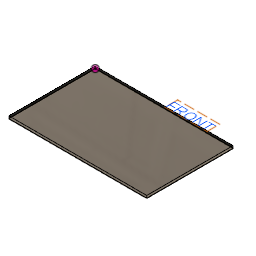
Irrigation unit - Solar panel (ZW 110x69) v3 (Autodesk Fusion 360 design; units mm, degrees)
Autodesk Fusion 360 part; units mm, degrees
sketch "Sketch1" plane through (0, 0, 0) normal (0, 0, 1) x (1, 0, 0)
  line L0 (0, 0) -> (110, 0)
  line L1 (110, 0) -> (110, -69)
  line L2 (110, -69) -> (0, -69)
  line L3 (0, -69) -> (0, 0)
  line L4 (54.46, 1.171) -> (87.8779, 1.171) construction
  line L5 (87.8779, 1.171) -> (87.8779, 11.171) construction
  line L6 (87.8779, 11.171) -> (54.46, 11.171) construction
  line L7 (54.46, 11.171) -> (54.46, 1.171) construction
  dimension "d1" = 69
  dimension "d2" = 110
extrude "Extrude1" add sketch "Sketch1" along normal blind 2
